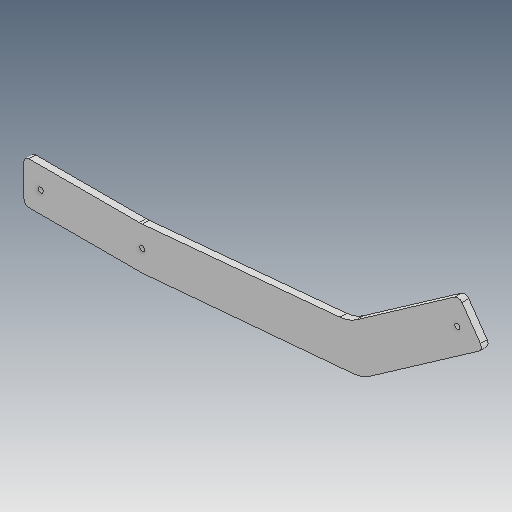
# Autodesk Inventor part: Träger vorne unten geknickt
Saved by Autodesk Inventor 2020 (Build 240168000, 168)
## iProperties
Created: 2021-06-29
Part Number: Träger vorne unten geknickt
Material: Generisch
Document SubType Name: Modeling
Designer: Mike
Density: 1 g/cm^3
Appearance: Vorgabe
Author: Mike
Autodesk Inventor part; units mm, degrees
ref_plane "YZ Plane" through (0, 0, 0) normal (1, 0, 0) x (0, 1, 0)
ref_plane "XZ Plane" through (0, 0, 0) normal (0, 1, 0) x (-1, 0, 0)
ref_plane "XY Plane" through (0, 0, 0) normal (0, 0, 1) x (1, 0, 0)
sketch "Skizze1" plane through (0, 0, 0) normal (0, 0, 1) x (1, 0, 0)
  line L0 (-147.1517, 0) -> (233.6885, 0) projected
  line L1 (0, -28.9385) -> (0, 86.5246) projected
  line L2 (-92.1246, 10.1776) -> (-92.1246, -8.8224)
  line L3 (-89.1246, -11.8224) -> (-22.9978, -11.8224)
  line L4 (-21.2547, -11.7463) -> (102.5368, -0.916)
  line L5 (112.2652, 2.6249) -> (176.8253, 47.8304)
  line L6 (177.562, 52.0085) -> (166.6641, 67.5724)
  line L7 (162.4859, 68.3092) -> (104.2561, 27.5362)
  line L8 (-89.1246, 13.1776) -> (-23.9199, 13.1776)
  line L9 (-22.0868, 13.2617) -> (94.6177, 24.0034)
  arc A0 (-22.9978, -11.8224) -> (-21.2547, -11.7463) centre (-22.9978, 8.1776) ccw
  arc A1 (102.5368, -0.916) -> (112.2652, 2.6249) centre (100.7937, 19.0079) ccw
  arc A2 (94.6177, 24.0034) -> (104.2561, 27.5362) centre (92.7846, 43.9193) ccw
  arc A3 (-23.9199, 13.1776) -> (-22.0868, 13.2617) centre (-23.9199, 33.1776) ccw
  arc A4 (-89.1246, 13.1776) -> (-92.1246, 10.1776) centre (-89.1246, 10.1776) ccw
  arc A5 (-92.1246, -8.8224) -> (-89.1246, -11.8224) centre (-89.1246, -8.8224) ccw
  arc A6 (176.8253, 47.8304) -> (177.562, 52.0085) centre (175.1046, 50.2878) ccw
  arc A7 (166.6641, 67.5724) -> (162.4859, 68.3092) centre (164.2066, 65.8517) ccw
  point P0 (0, 0)
  point P1 (-92.1246, 13.1776)
  point P2 (-92.1246, -11.8224)
  point P3 (-22.1246, -11.8224)
  point P4 (107.8754, -0.4489)
  point P5 (179.2828, 49.5511)
  point P6 (164.9434, 70.0299)
  dimension "d0" = 25
  dimension "d1" = 25
  dimension "d4" = 70
  dimension "d5" = 175
  dimension "d6" = 130
  dimension "d7" = 150
  dimension "d8" = 50
  dimension "d9" = 20
  dimension "d10" = 0.259
  dimension "d13" = 3
  constraints: 16 end point, 16 point on circle, 16 tangent, 12 point on line, 8 centre point, 6 equal radius, 3 perpendicular, 1 horizontal, 1 vertical
  measures "d0" distance of point (-92.125, 13.178) point (-92.125, -11.822)
  measures "d1" distance between parallel lines of L5 L7
  measures "d4" distance of point (-92.125, -11.822) point (-22.125, -11.822)
  measures "d5" angle of L3 L4
  measures "d6" horizontal distance of point (-22.125, -11.822) point (107.875, -0.449)
  measures "d7" angle of L5 L4
  measures "d8" vertical distance of point (107.875, -0.449) point (179.283, 49.551)
  measures "d9" radius of A0
  measures "d10" angle of L4 L9
  measures "d13" radius of A4
extrude "Extrusion1" add sketch "Skizze1" along normal blind 4
sketch "Skizze2" plane through (0, 0, 4) normal (0, 0, 1) x (1, 0, 0)
  line L0 (-23.9199, 13.1776) -> (-89.1246, 13.1776) projected
  line L1 (-92.1246, 10.1776) -> (-92.1246, -8.8224) projected
  line L2 (177.562, 52.0085) -> (166.6641, 67.5724) projected
  line L3 (112.2652, 2.6249) -> (176.8253, 47.8304) projected
  point P0 (0, 0)
  point P1 (-82.1246, 0.6776)
  point P2 (-22.1246, 0.6776)
  point P3 (163.9215, 54.0547)
  dimension "d14" = 12.5
  dimension "d15" = 10
  dimension "d16" = 60
  dimension "d17" = 12.5
  dimension "d18" = 10
  dimension "d19" = 12.5
  measures "d14" distance from line of L0 point (-82.125, 0.678)
  measures "d15" distance from line of L1 point (-82.125, 0.678)
  measures "d16" distance of point (-82.125, 0.678) point (-22.125, 0.678)
  measures "d17" distance from line of L0 point (-22.125, 0.678)
  measures "d18" distance from line of L2 point (163.922, 54.055)
  measures "d19" distance from line of L3 point (163.922, 54.055)
hole "Bohrung1" at (-82.1246, 0.6776, 4) at (-22.1246, 0.6776, 4) at (163.9215, 54.0547, 4) direction (0, 0, -1) diameter 3 depth 57.1 tip angle 118
